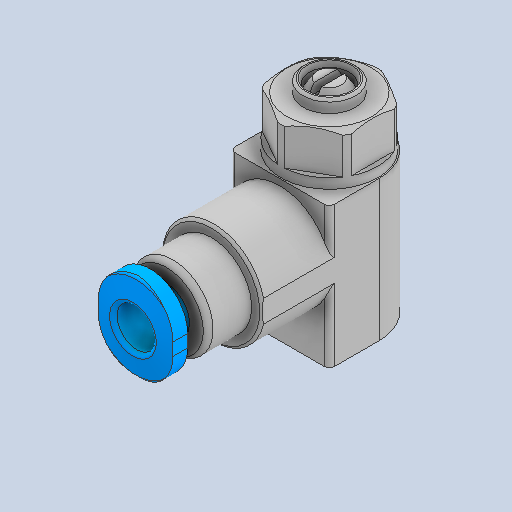
# Autodesk Inventor part: 175043 GRLZ-M3-QS-3
Saved by Autodesk Inventor 2025.2 (Build 292293000, 293)
## iProperties
Category: PARTsolutions
Company: FESTO
Created: 2025-06-16
Part Number: 175043 GRLZ-M3-QS-3
Material: Generic
Catalog Web Link: www.cadenas.de
Description: GRLZ-..-QS--(2)-one-way flow control valve
Vendor: FESTO
Document SubType Name: Modeling
Designer: psAdmin
Manufacturer: FESTO
Mass: 7 g
Surface Area: 10.5195 cm^2
Volume: 1.20545 cm^3
Density: 1 g/cm^3
Appearance: PSOLRGB-175-175-175
PSOL_IDENT_0: {$CADENAS_DATA/23d-libs/festo/parts/g/grlz/grlz_qs2.prj},187 {VTYP=3D},{NB=175043 GRLZ-M3-QS-3},{LIN
PSOL_IDENT_1: A=175043 GRLZ-M3-QS-3},{NN=GRLZ-..-QS--(2)},{DATE=22.08.2023 08:15:38},{GEOMDATE=22.08.2023 07:21:00
PSOL_IDENT_2: },{VERSION=},{LINEID=20},{WBVAR=},{WBNUMERIC=}  {NB=175043 GRLZ-M3-QS-3},{LINA=175043 GRLZ-M3-QS-3},
PSOL_IDENT_3: {KT=2},{TNR=175043},{TYP=GRLZ-M3-QS-3},{INFO=},{FORM=2},{D=M3},{D1=3.000},{D2=8.000},{BA=GRLZ},{DMM=
PSOL_IDENT_4: 3.000},{DKDR=2.387},{B=8.000},{B1=0.000},{L=16.600},{L1=2.300},{L2=7.000},{SW=7.000},{S=0.000},{H=20
PSOL_IDENT_5: .000},{H1=15.800},{T=1.000},{QS=3.000},{QSD=6.000},{DNC=0.000},{ZZ=0},{LHT=1.000},{WTS=0.600},{LTS=1
PSOL_IDENT_6: .960},{RSJ=4.000},{CHSJ=0.200},{HSJ=11.300},{RSJ1=0.400},{RSJ2=0.400},{DSJ=8.200},{LSJ=6.000},{LHSJ=
PSOL_IDENT_7: 5.500},{LQS=11.300},{LIQS=8.600},{DQS=6.500},{LIQS1=0.500},{LIQS2=0.000},{DHP=6.000},{DHP1=0.500},{D
PSOL_IDENT_8: NP=3.700},{LHP=1.400},{DHQS=3.150},{DR=4.800},{TR=0.300},{DBT=4.200},{DCH=6.800},{DH=7.800},{HHB=5.0
PSOL_IDENT_9: 00},{HH=4.200},{DI=1.500},{DIH=3.200},{LIH=0.400},{DR1=0.000},{DR2=0.000},{TR1=0.000},{LTR=0.000},{T
PSOL_IDENT_10: QS=9.500},{EOLDATE=},{CNSMASSEXACT=0.007},{ZOLL=3},{GTIN=4052568037673}
NB: 175043 GRLZ-M3-QS-3
NN: GRLZ-..-QS--(2)
NT: one-way flow control valve
NBSYN: $TNR. $TYP.
LINA: 175043 GRLZ-M3-QS-3
CATALOG: Festo
TNR: 175043
TYP: GRLZ-M3-QS-3
D: M3
D1: 3
D2: 8
B: 8
B1: 0
L: 16.6
L1: 2.3
L2: 7
SW: 7
S: 0
H: 20
H1: 15.8
T: 1
QS: 3
CNSMASSEXACT: 0.007
GTIN: 4052568037673
SUPPLIER: FESTO
ARTICLENO: 175043 GRLZ-M3-QS-3
BOMINFO: 175043 GRLZ-M3-QS-3
CREATOR: CADENAS GmbH
Title: 175043 GRLZ-M3-QS-3
Author: Cadenas PARTsolutions
Comments: one-way flow control valve
Autodesk Inventor part; units mm, degrees
sketch "Sketch_4" plane through (0, 0, 0) normal (1, 0, 0) x (0, 1, 0)
  line L0 (11.3, 0) -> (16.6, 0)
  line L1 (16.6, 0) -> (16.6, -0.98)
  line L2 (16.6, -0.98) -> (15.6, -1.6)
  line L3 (15.6, -1.6) -> (16.2, -1.6)
  line L4 (16.2, -1.6) -> (16.6, -1.7865)
  line L5 (16.6, -1.7865) -> (16.6, -1.9)
  line L6 (16.6, -1.9) -> (16.4, -2.1)
  line L7 (16.4, -2.1) -> (15.6, -2.1)
  line L8 (15.6, -2.1) -> (15.6, -3.4)
  line L9 (15.6, -3.4) -> (15.3113, -3.9)
  line L10 (15.3113, -3.9) -> (11.6, -3.9)
  line L11 (11.6, -3.9) -> (11.6, -2.4)
  line L12 (11.6, -2.4) -> (0, -2.4)
  line L13 (0, -2.4) -> (0, -1.5)
  line L14 (0, -1.5) -> (-1.9935, -1.5)
  line L15 (-1.9935, -1.5) -> (-2.3, -1.1935)
  line L16 (-2.3, -1.1935) -> (-2.3, -0.8655)
  line L17 (-2.3, -0.8655) -> (-2.1, -0.75)
  line L18 (-2.1, -0.75) -> (11.3, -0.75)
  line L19 (11.3, -0.75) -> (11.3, 0)
  line L20 (11.3, 0) -> (16.6, 0)
  constraints: 42 end point
revolve "Revolution1" add sketch "Sketch_4" angle 360 about axis through (0, 11.3, 0) along (0, 1, 0)
thread "Thread1" size "M3x0.5" class "6g" standard "ISO Metric profile" full length
sketch "Sketch_12" plane through (0, 0.3, 0) normal (0, 1, 0) x (1, 0, 0)
  arc A0 (-4, -3.6) -> (-3.6, -4) centre (-3.6, -3.6) ccw
  line L0 (-3.6, -4) -> (3.6, -4)
  arc A1 (3.6, -4) -> (4, -3.6) centre (3.6, -3.6) ccw
  line L1 (4, -3.6) -> (4, 0)
  arc A2 (4, 0) -> (-4, 0) centre (0, 0) ccw
  line L2 (-4, 0) -> (-4, -3.6)
  circle A3 centre (0, 0) radius 0.75
  constraints: 6 end point, 6 point on circle, 4 centre point
extrude "Extrusion1" add sketch "Sketch_12" along normal blind 11.3
sketch "Sketch_13" plane through (0, 0, 0) normal (1, 0, 0) x (0, 1, 0)
  line L0 (7, 3.5) -> (7, 6.3)
  line L1 (7, 6.3) -> (8.575, 6.3)
  line L2 (8.575, 6.3) -> (8.575, 15.5)
  arc A0 (8.875, 15.8) -> (8.575, 15.5) centre (8.875, 15.5) ccw
  line L3 (8.875, 15.8) -> (10.3347, 15.5426)
  arc A1 (10.5, 15.3456) -> (10.3347, 15.5426) centre (10.3, 15.3456) ccw
  line L4 (10.5, 15.3456) -> (10.5, 14.4)
  line L5 (10.5, 14.4) -> (9.05, 14.4)
  arc A2 (9.05, 14.4) -> (8.85, 14.2) centre (9.05, 14.2) ccw
  line L6 (8.85, 14.2) -> (8.85, 13.1)
  line L7 (8.85, 13.1) -> (9.9613, 13.1)
  line L8 (9.9613, 13.1) -> (10.25, 12.6)
  line L9 (10.25, 12.6) -> (10.25, 9.5)
  line L10 (10.25, 9.5) -> (10.9, 9.5)
  line L11 (10.9, 9.5) -> (11.1, 9.3)
  line L12 (11.1, 9.3) -> (11.1, 3.5)
  line L13 (11.1, 3.5) -> (7, 3.5)
  line L14 (7, 3.5) -> (7, 6.3)
  constraints: 30 end point, 6 point on circle, 3 centre point
revolve "Revolution2" add sketch "Sketch_13" angle 360 about axis through (0, 7, 3.5) along (0, 0, -1)
sketch "Sketch_14" plane through (0, 16.6, 0) normal (0, 1, 0) x (1, 0, 0)
  line L0 (-5, -6) -> (5, -6)
  line L1 (5, -6) -> (5, 6)
  line L2 (5, 6) -> (-5, 6)
  line L3 (-5, 6) -> (-5, -6)
  line L4 (-3.5, -2.0207) -> (0, -4.0415)
  line L5 (0, -4.0415) -> (3.5, -2.0207)
  line L6 (3.5, -2.0207) -> (3.5, 2.0207)
  line L7 (3.5, 2.0207) -> (0, 4.0415)
  line L8 (0, 4.0415) -> (-3.5, 2.0207)
  line L9 (-3.5, 2.0207) -> (-3.5, -2.0207)
  constraints: 20 end point
extrude "Extrusion2" cut sketch "Sketch_14" against normal blind 4.2
sketch "Sketch_15" plane through (0, 16.6, 0) normal (0, 1, 0) x (1, 0, 0)
  line L0 (-0.3, 1.5207) -> (-0.3, -1.5207)
  arc A0 (-0.3, -1.5207) -> (0.3, -1.5207) centre (0, 0) ccw
  line L1 (0.3, -1.5207) -> (0.3, 1.5207)
  arc A1 (0.3, 1.5207) -> (-0.3, 1.5207) centre (0, 0) ccw
  constraints: 4 end point, 4 point on circle, 2 centre point
extrude "Extrusion3" cut sketch "Sketch_15" against normal blind 0.8
sketch "Sketch_16" plane through (0, 0, 0) normal (0, 0, 1) x (1, 0, 0)
  line L0 (-9, 35) -> (-9, -15)
  line L1 (-9, -15) -> (9, -15)
  line L2 (9, -15) -> (9, 35)
  line L3 (9, 35) -> (-9, 35)
  line L4 (-4, 31.6) -> (-4, -10)
  line L5 (-4, -10) -> (4, -10)
  line L6 (4, -10) -> (4, 31.6)
  line L7 (4, 31.6) -> (-4, 31.6)
  constraints: 16 end point
extrude "Extrusion4" cut sketch "Sketch_16" along normal blind 15.8
sketch "Sketch_7" plane through (0, 0, 0) normal (1, 0, 0) x (0, 1, 0)
  line L0 (7, 0) -> (7, 15.8)
  line L1 (7, 15.8) -> (8.8, 15.8)
  arc A0 (8.8, 15.8) -> (8.5, 15.5) centre (8.8, 15.5) ccw
  line L2 (8.5, 15.5) -> (8.5, 6.3)
  line L3 (8.5, 6.3) -> (7.75, 6.3)
  line L4 (7.75, 6.3) -> (7.75, 0)
  line L5 (7.75, 0) -> (7, 0)
  line L6 (7, 0) -> (7, 15.8)
  constraints: 14 end point, 2 point on circle, 1 centre point
revolve "Revolution3" cut sketch "Sketch_7" angle 360 about axis through (0, 7, 0) along (0, 0, -1)
sketch "Sketch_17" plane through (0, 0, 15.8) normal (0, 0, 1) x (1, 0, 0)
  line L0 (-6.7662, -4.0731) -> (6.559, -4.0731)
  line L1 (6.559, -4.0731) -> (6.559, 17.5987)
  line L2 (6.559, 17.5987) -> (-6.7662, 17.5987)
  line L3 (-6.7662, 17.5987) -> (-6.7662, -4.0731)
  arc A0 (-3, 6.5) -> (3, 6.5) centre (0, 6.5) ccw
  line L4 (3, 6.5) -> (3, 7.5)
  arc A1 (3, 7.5) -> (-3, 7.5) centre (0, 7.5) ccw
  line L5 (-3, 7.5) -> (-3, 6.5)
  constraints: 12 end point, 4 point on circle, 2 centre point
extrude "Extrusion5" cut sketch "Sketch_17" against normal blind 1.4
ref_plane "FDT_MOUNT_XY" through (0, 0, 0) normal (0, 1, 0) x (-1, 0, 0)
ref_plane "FDT_MOUNT_YZ" through (0, 0, 0) normal (-1, 0, 0) x (0, 0, 1)
ref_plane "FDT_MOUNT_ZX" through (0, 0, 0) normal (0, 0, 1) x (0, 1, 0)
ref_plane "FDT_SCHLAUCH_XY" through (0, 7, 6.3) normal (0, 0, 1) x (1, 0, 0)
ref_plane "FDT_SCHLAUCH_YZ" through (0, 7, 6.3) normal (1, 0, 0) x (0, 1, 0)
ref_plane "FDT_SCHLAUCH_ZX" through (0, 7, 6.3) normal (0, 1, 0) x (0, 0, 1)
ref_plane "Schlauch_XY" through (0, 7, 15.8) normal (0, 0, 1) x (1, 0, 0)
ref_plane "Schlauch_YZ" through (0, 7, 15.8) normal (1, 0, 0) x (0, 1, 0)
ref_plane "Schlauch_ZX" through (0, 7, 15.8) normal (0, 1, 0) x (0, 0, 1)
ref_plane "Zylinder_XY" through (0, -2.3, 0) normal (0, 1, 0) x (1, 0, 0)
ref_plane "Zylinder_YZ" through (0, -2.3, 0) normal (1, 0, 0) x (0, 0, -1)
ref_plane "Zylinder_ZX" through (0, -2.3, 0) normal (0, 0, -1) x (0, 1, 0)
ref_plane "anbau_XY" through (0, 0, 0) normal (0, 1, 0) x (1, 0, 0)
ref_plane "anbau_YZ" through (0, 0, 0) normal (1, 0, 0) x (0, 0, -1)
ref_plane "anbau_ZX" through (0, 0, 0) normal (0, 0, -1) x (0, 1, 0)
body "Solid1"
